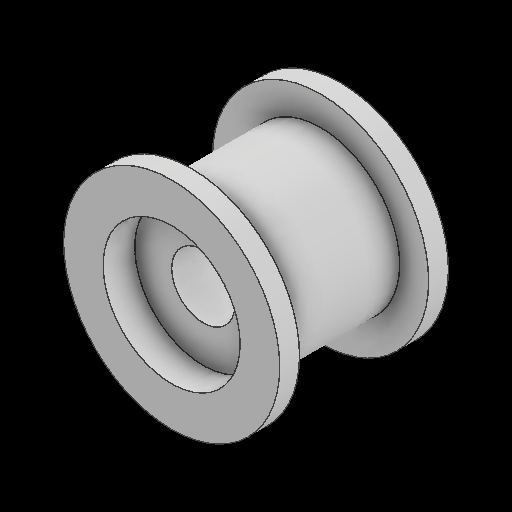
# Autodesk Inventor part: LegChainTensionerBlock
Saved by Autodesk Inventor 2025.2 (Build 292293000, 293)
## iProperties
Created: 2026-01-19
Part Number: LegChainTensionerBlock
Material: Generic
Document SubType Name: Modeling
Designer: valer
Density: 1 g/cm^3
Appearance: Default
Author: valer
Autodesk Inventor part; units mm, degrees
ref_plane "YZ Plane" through (0, 0, 0) normal (1, 0, 0) x (0, 1, 0)
ref_plane "XZ Plane" through (0, 0, 0) normal (0, 1, 0) x (-1, 0, 0)
ref_plane "XY Plane" through (0, 0, 0) normal (0, 0, 1) x (1, 0, 0)
sketch "Base" plane through (0, 0, 0) normal (0, 0, 1) x (1, 0, 0)
  circle A0 centre (0, 0) radius 10.25
  dimension "d0" = 20.5
  constraints: 1 centre point, 1 coincident
  measures "d0" diameter of A0
extrude "BaseFeature" add sketch "Base" along normal mid plane 16
sketch "Ridges" plane through (0, 0, 0) normal (0, 0, 1) x (1, 0, 0)
  circle A0 centre (0, 0) radius 10.25 projected
  circle A1 centre (0, 0) radius 7.5
  dimension "d3" = 15
  constraints: 1 centre point, 1 coincident
  measures "d3" diameter of A1
extrude "RidgesFeature" cut sketch "Ridges" along normal mid plane 12.25
sketch "Countersink" plane through (0, 0, 8) normal (0, 0, 1) x (1, 0, 0)
  circle A0 centre (0, 0) radius 6.5
  dimension "d6" = 13
  constraints: 1 centre point, 1 coincident
  measures "d6" diameter of A0
extrude "CountersinkFeature" cut sketch "Countersink" against normal blind 3
mirror "CountersinkMirrorFeature" about plane through (0, 0, 0) normal (0, 0, 1) of "CountersinkFeature"
sketch "MountHole" plane through (0, 0, 5) normal (0, 0, 1) x (1, 0, 0)
  point P0 (0, 0)
hole "MountHoleFeature" at (0, 0, 5) direction (0, 0, -1) diameter 6 end through all
body "Solid1"
